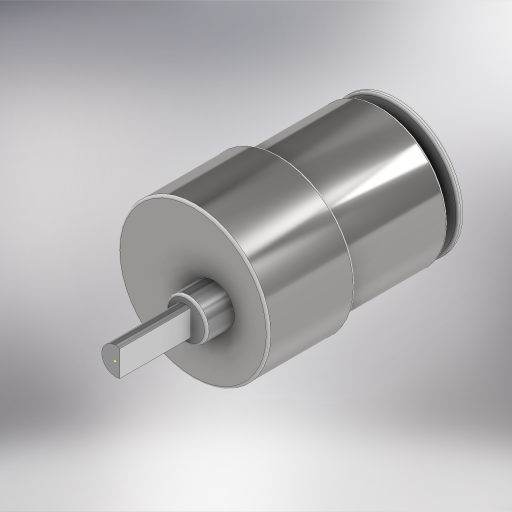
# Autodesk Inventor part: Motor
Saved by Autodesk Inventor 2024 (Build 280153000, 153)
## iProperties
Created: 2023-11-01
Part Number: Motor
Material: Genérico
Document SubType Name: Modeling
Designer: juesr
Density: 1 g/cm^3
Appearance: Valor por defecto
Author: juesr
Autodesk Inventor part; units mm, degrees
ref_plane "YZ Plane" through (0, 0, 0) normal (1, 0, 0) x (0, 1, 0)
ref_plane "XZ Plane" through (0, 0, 0) normal (0, 1, 0) x (-1, 0, 0)
ref_plane "XY Plane" through (0, 0, 0) normal (0, 0, 1) x (1, 0, 0)
sketch "Boceto1" plane through (0, 0, 0) normal (0, 0, 1) x (1, 0, 0)
  circle A0 centre (0, 0) radius 3
  dimension "d0" = 6
  constraints: 1 centre point, 1 coincident
  measures "d0" diameter of A0
extrude "Extrusión1" add sketch "Boceto1" along normal blind 15.5
sketch "Boceto2" plane through (0, 0, 0) normal (0, 0, -1) x (-1, 0, 0)
  circle A0 centre (0, 0) radius 4.5
  dimension "d3" = 9
  constraints: 1 centre point, 1 coincident
  measures "d3" diameter of A0
extrude "Extrusión2" add sketch "Boceto2" along normal blind 6
sketch "Boceto3" plane through (0, 0, 15.5) normal (0, 0, 1) x (1, 0, 0)
  point P0 (0, 0)
sketch "Boceto4" plane through (0, 0, -6) normal (0, 0, -1) x (-1, 0, 0)
  point P0 (0, 0)
sketch "Boceto5" plane through (0, 0, 15.5) normal (0, 0, 1) x (1, 0, 0)
  line L0 (1, 3.0944) -> (7.331, 3.0944)
  line L1 (7.331, 3.0944) -> (7.331, -4.1969)
  line L2 (7.331, -4.1969) -> (1, -4.1969)
  line L3 (1, -4.1969) -> (1, 3.0944)
  point P0 (0, 0)
  dimension "d6" = 1
  constraints: 8 end point, 2 parallel, 1 horizontal, 1 perpendicular
  measures "d6" distance from line of point (0, 0) L3
extrude "Extrusión3" cut sketch "Boceto5" against normal blind 15.5
sketch "Boceto6" plane through (0, 0, -6) normal (0, 0, -1) x (-1, 0, 0)
  circle A0 centre (4.5, 0) radius 16.5
  point P0 (0, 0)
  dimension "d9" = 4.5
  dimension "d10" = 33
  constraints: 1 centre point
  measures "d9" distance of point (0, 0) A0.centre
  measures "d10" diameter of A0
extrude "Extrusión4" add sketch "Boceto6" along normal blind 19
sketch "Boceto7" plane through (-4.5, 0, -25) normal (0, 0, -1) x (-1, 0, 0)
  circle A0 centre (-4.5, 0) radius 4.5 projected
  circle A1 centre (0, 0) radius 14.75
  dimension "d13" = 29.5
  constraints: 1 centre point, 1 horizontal alignment, 1 other
  measures "d13" diameter of A1
extrude "Extrusión5" add sketch "Boceto7" along normal blind 22 contours A0 | A1
sketch "Boceto8" plane through (-4.5, 0, -47) normal (0, 0, -1) x (-1, 0, 0)
  circle A0 centre (-4.5, 0) radius 4.5 projected
  circle A1 centre (0, 0) radius 5
  dimension "d16" = 10
  constraints: 1 centre point, 1 horizontal alignment, 1 other
  measures "d16" diameter of A1
extrude "Extrusión6" add sketch "Boceto8" along normal blind 2.5 contours A0 A1 | A0 A1 picked at (-3.3248, -0.7551) picked at (3.2856, 0.3961)
sketch "Boceto9" plane through (-4.5, 0, -49.5) normal (0, 0, -1) x (-1, 0, 0)
  circle A0 centre (-4.5, 0) radius 4.5 projected
  circle A1 centre (0, 0) radius 14.5
  constraints: 1 centre point, 1 horizontal alignment, 1 other
extrude "Extrusión7" add sketch "Boceto9" along normal blind 1.5 contours A0 | A1
sketch "Boceto10" plane through (-4.5, 0, -51) normal (0, 0, -1) x (-1, 0, 0)
  circle A0 centre (-4.5, 0) radius 4.5 projected
  circle A1 centre (0, 0) radius 7.5
  dimension "d21" = 15
  constraints: 1 centre point, 1 horizontal alignment, 1 other
  measures "d21" diameter of A1
extrude "Extrusión8" add sketch "Boceto10" along normal blind 4 contours A0 A1 | A0 A1 picked at (-4.9657, 0) picked at (4.9328, -0.5757)
fillet "Empalme1" radius 0.5 1 edges at (4.5, 0, 0)
fillet "Empalme2" radius 0.5 1 edges at (12, 0, -6)
fillet "Empalme3" radius 0.5 1 edges at (12, 0, -25)
fillet "Empalme4" radius 0.5 1 edges at (10.25, 0, -47)
fillet "Empalme5" radius 0.5 1 edges at (10, 0, -49.5)
fillet "Empalme6" radius 0.5 1 edges at (10, 0, -51)
fillet "Empalme7" radius 1 1 edges at (3, 0, -55)
